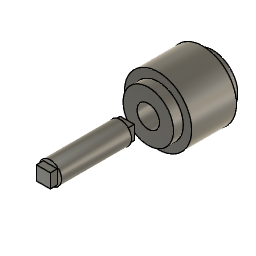
Anvil DIe and The Mount (Autodesk Fusion 360 design; units mm, degrees)
Autodesk Fusion 360 part; units mm, degrees
sketch "Sketch1" plane through (0, 0, 0) normal (0, 1, 0) x (1, 0, 0)
  line L0 (3.175, 3.175) -> (-3.175, 3.175)
  line L1 (-3.175, 3.175) -> (-3.175, -3.175)
  line L2 (-3.175, -3.175) -> (3.175, -3.175)
  line L3 (3.175, -3.175) -> (3.175, 3.175)
  dimension "d1" = 6.35
  dimension "d2" = 6.35
  constraint horizontal L0
  constraint perpendicular L0 L1
  constraint parallel L0 L2
  constraint parallel L1 L3
  measures "d1" distance of L1.end L2.end
  measures "d2" distance of L0.end L1.end
extrude "Extrude1" add sketch "Sketch1" along normal blind 38.1 makes body 1
sketch "Sketch2" plane through (0, 0, 0) normal (0, 1, 0) x (1, 0, 0)
move_body "Move1" bodies 1 to x (1, 0, 0) y (0, 1, 0) z (0, 0, 1) at (0, -19.05, 0)
sketch "Sketch3" plane through (0, 0, 0) normal (0, 1, 0) x (1, 0, 0)
  circle A0 centre (0, 0) radius 3.81
  circle A1 centre (0, 0) radius 5.5938
  dimension "d6" = 7.62
  constraint coincident A0.centre A1.centre
  constraint concentric A0 A1
  measures "d6" diameter of A0
sketch "Sketch4" plane through (0, 0, 0) normal (0, 1, 0) x (1, 0, 0)
  circle A0 centre (0, 0) radius 5.08
  constraint coincident A0.centre origin
extrude "Extrude4" add sketch "Sketch4" along normal blind 15.875 and the other way blind 15.875 bodies 1
copy_body "Body->Comp1" bodies 1 removing the originals makes body 2 in component "Mount"
sketch "Sketch5" plane through (0, 0, 0) normal (0, 1, 0) x (1, 0, 0)
  circle A0 centre (0, 0) radius 5.08
  circle A1 centre (0, 0) radius 15.24
  dimension "d19" = 10.16
  dimension "d20" = 30.48
  constraint coincident A0.centre A1.centre
  constraint concentric A0 A1
  measures "d19" diameter of A0
  measures "d20" diameter of A1
extrude "Extrude5" add sketch "Sketch5" along normal blind 25.4 separate body makes body 3
sketch "Sketch6" plane through (0, 25.4, 0) normal (0, 1, 0) x (-1, 0, 0)
  circle A0 centre (0, 0) radius 5.08
  circle A1 centre (0, 0) radius 15.24
  circle A2 centre (0, 0) radius 11.43
  dimension "d23" = 22.86
  constraint coincident A0.centre A1.centre
  measures "d23" diameter of A2
sketch "Sketch7" plane through (0, 25.4, 0) normal (0, 1, 0) x (-1, 0, 0)
sketch "Sketch8" plane through (0, 0, 0) normal (0, -1, 0) x (1, 0, 0)
  circle A0 centre (0, 0) radius 5.08
  circle A1 centre (0, 0) radius 15.24
  circle A2 centre (0, 0) radius 11.43
  dimension "d25" = 22.86
  constraint concentric A0 A2
  measures "d25" diameter of A2
extrude "Extrude6" cut sketch "Sketch6" against normal blind 2.54 contours A1 bodies 3
extrude "Extrude7" cut sketch "Sketch8" against normal blind 2.54 contours A1 bodies 3
copy_body "Body->Comp2" bodies 3 removing the originals makes body 4 in component "Anvil Die"
extrude "Extrude1'" add 1 faces at (9.2519, 0, -0.8202) along direction (0, -1, 0) blind 1.905 on bodies 4 bodies 4 in component "Anvil Die"
extrude "Extrude2" add 1 faces at (-9.2519, 25.4, -0.8202) along direction (0, 1, 0) blind 1.905 on bodies 4 bodies 4 in component "Anvil Die"
component "Mount" placed x (1, 0, 0) y (0, 1, 0) z (0, 0, 1) at (0, 0, 0)
component "Anvil Die" placed x (1, 0, 0) y (0, 1, 0) z (0, 0, 1) at (0, 0, 0)
named bodies: "Mount", "Anvil Die"
